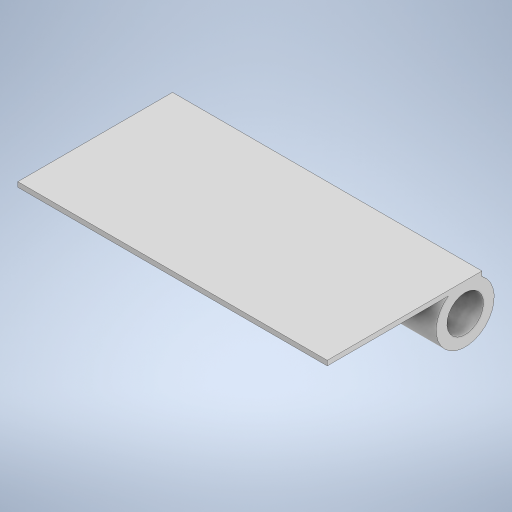
# Autodesk Inventor part: AxleHolder
Saved by Autodesk Inventor 2023.4 (Build 274418000, 418)
## iProperties
Created: 2026-03-03
Part Number: AxleHolder
Material: Generic
Document SubType Name: Modeling
Designer: 1017208
Density: 1 g/cm^3
Appearance: Default
Author: 1017208
Autodesk Inventor part; units mm, degrees
ref_plane "YZ Plane" through (0, 0, 0) normal (1, 0, 0) x (0, 1, 0)
ref_plane "XZ Plane" through (0, 0, 0) normal (0, 1, 0) x (-1, 0, 0)
ref_plane "XY Plane" through (0, 0, 0) normal (0, 0, 1) x (1, 0, 0)
sketch "Sketch1" plane through (0, 0, 0) normal (1, 0, 0) x (0, 1, 0)
  circle A0 centre (0, 0) radius 3
  circle A1 centre (0, 0) radius 4.7625
  line L0 (4.7625, 0) -> (3, 0)
  line L1 (3.8813, 0) -> (3.8813, 2.7599)
  line L2 (3.8813, 0) -> (3.8813, -2.7599)
  dimension "d0" = 6
  constraints: 6 end point, 3 point on circle, 1 centre point, 1 coincident, 1 horizontal, 1 horizontal alignment, 1 midpoint, 1 point on line, 1 vertical, 2 other
extrude "Extrusion1" add sketch "Sketch1" against normal blind 50.8 contours L1 L2 A1
sketch "Sketch2" plane through (0, 3.8813, 2.7599) normal (0, 1, 0) x (1, 0, 0)
  line L0 (0, 5.5199) -> (-50.8, 5.5199) projected
  line L1 (0, 5.5199) -> (-50.8, 5.5199)
  line L2 (-50.8, 5.5199) -> (-50.8, -19.8801)
  line L3 (-50.8, -19.8801) -> (0, -19.8801)
  line L4 (0, -19.8801) -> (0, 5.5199)
  point P0 (0, 0)
  dimension "d7" = 50.8
  dimension "d8" = 25.4
  constraints: 8 end point, 2 parallel, 1 horizontal, 1 perpendicular
  measures "d7" distance of L3.end L2.end
  measures "d8" distance of L2.end L1.end
extrude "Extrusion2" add sketch "Sketch2" along normal blind 0.7937
body "Solid1"
